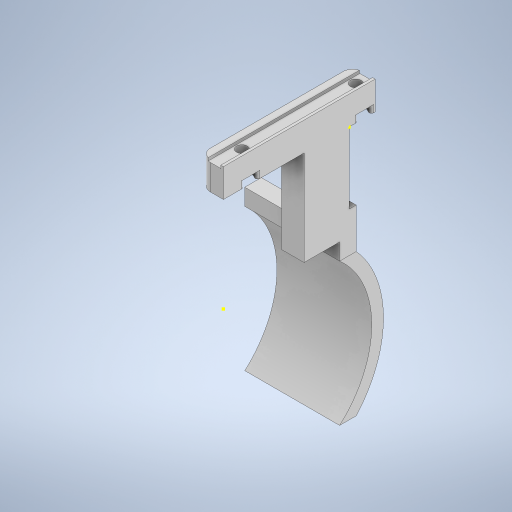
# Autodesk Inventor part: Back
Saved by Autodesk Inventor 2024 (Build 280153000, 153)
## iProperties
Created: 2023-12-18
Part Number: Back
Material: Generic
Document SubType Name: Modeling
Designer: Mechatronics Lab 1
Density: 1 g/cm^3
Appearance: Default
Author: Mechatronics Lab 1
Autodesk Inventor part; units mm, degrees
ref_plane "YZ Plane" through (0, 0, 0) normal (1, 0, 0) x (0, 1, 0)
ref_plane "XZ Plane" through (0, 0, 0) normal (0, 1, 0) x (-1, 0, 0)
ref_plane "XY Plane" through (0, 0, 0) normal (0, 0, 1) x (1, 0, 0)
sketch "Sketch1" plane through (0, 0, 0) normal (0, 1, 0) x (-1, 0, 0)
  line L0 (0, 0) -> (9.5, 0)
  line L1 (9.5, 0) -> (9.5, -64)
  line L2 (9.5, -64) -> (0, -64)
  line L3 (0, -64) -> (0, 0)
  circle A0 centre (3.7, -11.5) radius 2.25
  circle A1 centre (3.7, -59.5) radius 2.25
  line L4 (3.7, -11.5) -> (3.7, -59.5) construction
  dimension "d1" = 9.5
  dimension "d2" = 64
  dimension "d3" = 4.5
  dimension "d4" = 48
  dimension "d6" = 3.7
  dimension "d17" = 4.5
  constraints: 10 end point, 2 centre point, 2 parallel, 1 equal radius, 1 horizontal, 1 perpendicular, 1 vertical
  measures "d1" distance of L0.start L0.end
  measures "d2" distance of L0.end L1.end
  measures "d3" diameter of A0
  measures "d4" distance of L4.start L4.end
  measures "d6" distance between parallel lines of L3 L4
  measures "d17" distance from line of L4.end L2
extrude "Extrusion1" add sketch "Sketch1" along normal blind 12
sketch "Sketch2" plane through (-9.5, 0, 0) normal (0, 0, 1) x (1, 0, 0)
  line L0 (9.5, 12) -> (0, 12) projected
  line L1 (3, 12) -> (8.4, 12)
  line L2 (8.4, 12) -> (8.4, 10.8)
  line L3 (8.4, 10.8) -> (3, 10.8)
  line L4 (3, 10.8) -> (3, 12)
  line L5 (9.5, 0) -> (9.5, 12) projected
  line L6 (3.55, 0) -> (8.05, 0) projected
  line L7 (3.55, 12) -> (8.05, 12) projected
  line L8 (9.5, 0) -> (9.5, 12) projected
  line L9 (9.5, 0) -> (9.5, 12) projected
  line L10 (3.55, 12) -> (8.05, 12) projected
  line L11 (3.55, 12) -> (3.55, 0) projected
  line L12 (3.55, 12) -> (8.05, 12) projected
  line L13 (3.55, 0) -> (8.05, 0) projected
  line L14 (3.55, 12) -> (8.05, 12) projected
  line L15 (3.55, 0) -> (8.05, 0) projected
  line L16 (3.55, 12) -> (8.05, 12) projected
  line L17 (3.55, 0) -> (8.05, 0) projected
  dimension "d9" = 1.1
  dimension "d10" = 5.4
  dimension "d11" = 1.2
  dimension "d76" = 12
  constraints: 8 end point, 2 parallel, 1 horizontal, 1 perpendicular, 1 point on line
  measures "d9" distance between parallel lines of L5 L2
  measures "d10" distance of L2.end L3.end
  measures "d11" distance between parallel lines of L0 L3
  measures "d76" distance between parallel lines of L6 L7
extrude "Extrusion2" cut sketch "Sketch2" against normal up to next
sketch "Sketch3" plane through (0, 0, 0) normal (0, -1, 0) x (1, 0, 0)
  circle A0 centre (-3.7, -11.5) radius 2.25 projected
  circle A1 centre (-3.7, -11.5) radius 3.75
  circle A2 centre (-3.7, -59.5) radius 2.25 projected
  circle A3 centre (-3.7, -59.5) radius 3.75
  point P0 (0, 0)
  dimension "d14" = 7.5
  constraints: 2 centre point, 2 coincident, 1 equal radius
  measures "d14" diameter of A3
extrude "Extrusion3" cut sketch "Sketch3" against normal blind 3
fillet "Fillet1" radius 1 4 edges at (0, 1.5, -58.8897) (0, 1.5, -60.1103) (0, 1.5, -10.8897) (0, 1.5, -12.1103)
fillet "Fillet2" radius 4 2 edges at (-9.5, 6, -64) (-9.5, 6, 0)
sketch "Sketch28" plane through (0, 0, 0) normal (0, -1, 0) x (1, 0, 0)
  arc A0 (-1.5684, -56.4147) -> (0, -55.592) centre (-1, -55.592) ccw projected
  line L0 (0, -55.592) -> (0, -53)
  line L1 (0, -15.408) -> (0, -55.592) projected
  line L2 (-9.5, -60) -> (-9.5, -4) projected
  line L3 (0, -53) -> (-9.5, -53)
  line L4 (-9.5, -53) -> (-9.5, -34)
  line L5 (-9.5, -34) -> (0, -34)
  line L6 (0, -34) -> (0, -53)
  point P0 (0, 0)
  point P1 (0, -34)
  dimension "d107" = 2.592
  dimension "d108" = 19
  constraints: 10 end point, 2 parallel, 2 point on line, 1 horizontal, 1 perpendicular
  measures "d107" distance of L0.start L0.end
  measures "d108" distance of L3.end L4.end
extrude "Extrusion19" add sketch "Sketch28" along normal blind 30
sketch "Sketch40" plane through (0, -30, 0) normal (0, -1, 0) x (1, 0, 0)
  line L0 (0, -53) -> (-9.5, -53) projected
  line L1 (-9.5, -53) -> (-9.5, -56)
  line L2 (-9.5, -56) -> (0, -56)
  line L3 (0, -56) -> (0, -34)
  line L4 (0, 0) -> (0, -64) projected
  line L5 (0, -34) -> (-9.5, -34)
  line L6 (-9.5, -34) -> (-9.5, -53)
  line L7 (-9.5, -34) -> (0, -34)
  line L8 (0, -34) -> (0, -56)
  line L9 (0, -56) -> (-9.5, -56)
  line L10 (-9.5, -56) -> (-9.5, -34)
  dimension "d130" = 3
  dimension "d131" = 22
  constraints: 18 end point, 3 perpendicular, 2 parallel, 2 point on line, 1 collinear, 1 horizontal, 1 vertical
  measures "d130" distance of L0.end L1.end
  measures "d131" distance of L2.end L3.end
extrude "Extrusion21" add sketch "Sketch40" along normal blind 10
sketch "Sketch41" plane through (0, 0, -53) normal (0, 0, -1) x (-1, 0, 0)
  point P0 (0, 0)
sketch "Sketch42" plane through (0, -40, 0) normal (0, -1, 0) x (1, 0, 0)
  line L0 (-9.5, -56) -> (0, -56) projected
  line L1 (-9.5, -56) -> (-40, -56)
  line L2 (-9.5, -56) -> (21, -56) construction
  line L3 (-40, -56) -> (-40, -49)
  line L4 (-40, -49) -> (0, -49)
  line L5 (0, -49) -> (0, -56)
  line L6 (0, -56) -> (-9.5, -56)
  point P0 (0, 0)
  point P1 (0, -56)
  dimension "d134" = 30.5
  dimension "d135" = 180
  dimension "d136" = 7
  dimension "d137" = 40
  dimension "d138" = 7
  constraints: 12 end point, 2 horizontal, 2 perpendicular, 1 collinear, 1 point on line
  measures "d134" distance of L0.start L1.end
  measures "d135" angle of L1 L2
  measures "d136" distance of L1.end L3.end
  measures "d137" distance of L3.end L4.end
  measures "d138" distance of L4.end L5.end
extrude "Extrusion22" add sketch "Sketch42" along normal blind 7
sketch "Sketch54" plane through (-40, -40, -56) normal (-1, 0, 0) x (0, 0, 1)
  arc A0 (7, -7) -> (7, -57) centre (31.4949, -32) ccw projected
  line L0 (-6.4428, -57) -> (19.2704, -57)
  line L1 (19.2704, -57) -> (19.2704, -74.6848)
  line L2 (19.2704, -74.6848) -> (-6.4428, -74.6848)
  line L3 (-6.4428, -74.6848) -> (-6.4428, -57)
  point P0 (56, 40)
  constraints: 8 end point, 2 parallel, 1 horizontal, 1 perpendicular
extrude "Extrusion25" cut sketch "Sketch54" against normal blind 104.3
sketch "Sketch56" plane through (0, -47, 0) normal (0, -1, 0) x (1, 0, 0)
  line L0 (-40, -56) -> (0, -56) projected
  line L1 (0, -56) -> (0, -49) projected
  line L2 (-40, -56) -> (0, -56)
  line L3 (0, -56) -> (0, -49)
  line L4 (0, -49) -> (-40, -49)
  line L5 (-40, -49) -> (-40, -56)
  point P0 (0, 0)
  point P1 (9.3, -58)
  constraints: 8 end point, 2 parallel, 1 horizontal, 1 perpendicular, 2 other
sketch "Sketch58" plane through (-40, -40, -56) normal (-1, 0, 0) x (0, 0, 1)
  arc A0 (7, -7) -> (7, -67) centre (33.4575, -37) ccw
  point P0 (56, 40)
  dimension "d164" = 60
  dimension "d165" = 40
  constraints: 2 point on circle, 1 centre point
  measures "d164" distance of A0.start A0.end
  measures "d165" radius of A0
sweep "Sweep4" add profiles "Sketch56" path "Sketch58" separate body
sketch "Sketch59" plane through (-40, -47, -56) normal (-1, 0, 0) x (0, 0, 1)
  line L0 (7.875, -66.9451) -> (7, -60) projected
  line L1 (7, -60) -> (-3.876, -60)
  line L2 (-3.876, -60) -> (-3.876, -70.2842)
  line L3 (-3.876, -70.2842) -> (7, -70.2842)
  line L4 (7, -70.2842) -> (7, -60)
  line L5 (-3.876, -60) -> (12.796, -60)
  line L6 (12.796, -60) -> (12.796, -72.0421)
  line L7 (12.796, -72.0421) -> (-3.876, -72.0421)
  line L8 (-3.876, -72.0421) -> (-3.876, -60)
  point P0 (56, 47)
  point P1 (7, -60)
  constraints: 16 end point, 4 parallel, 2 horizontal, 2 perpendicular
extrude "Extrusion26" cut sketch "Sketch59" against normal blind 63.025 bodies 2
sketch "Sketch60" plane through (0, -40, 0) normal (0, 1, 0) x (1, 0, 0)
  point P0 (0, 0)
body "Solid1"
body "Solid2"
